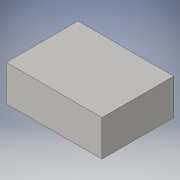
# Autodesk Inventor part: Brain
Saved by Autodesk Inventor 2016 (Build 200138000, 138)
## iProperties
Created: 2015-10-30
Part Number: Brain
Material: Generic
Document SubType Name: Modeling
Designer: rossmosier
Density: 1 g/cm^3
Appearance: Default
Author: rossmosier
Autodesk Inventor part; units mm, degrees
ref_plane "YZ Plane" through (0, 0, 0) normal (1, 0, 0) x (0, 1, 0)
ref_plane "XZ Plane" through (0, 0, 0) normal (0, 1, 0) x (-1, 0, 0)
ref_plane "XY Plane" through (0, 0, 0) normal (0, 0, 1) x (1, 0, 0)
sketch "Sketch1" plane through (0, 0, 0) normal (0, 1, 0) x (-1, 0, 0)
  line L0 (0, 0) -> (-203.2, 0)
  line L1 (-203.2, 0) -> (-203.2, -152.4)
  line L2 (-203.2, -152.4) -> (0, -152.4)
  line L3 (0, -152.4) -> (0, 0)
  dimension "d0" = 203.2
  dimension "d1" = 152.4
  constraints: 8 end point, 2 parallel, 1 horizontal, 1 perpendicular
  measures "d0" distance of L2.end L1.end
  measures "d1" distance of L1.end L0.end
extrude "Extrusion1" add sketch "Sketch1" along normal blind 76.2
sketch "Sketch2" plane through (0, 76.2, 0) normal (0, 1, 0) x (1, 0, 0)
  line L0 (0, 0) -> (203.2, 0) projected
  line L1 (203.2, 0) -> (203.2, 152.4) projected
  line L2 (203.2, 152.4) -> (0, 152.4) projected
  line L3 (0, 152.4) -> (0, 0) projected
  line L4 (203.2, 0) -> (101.6, 0) construction
  line L5 (101.6, 63.5) -> (203.2, 63.5) construction
  line L6 (203.2, 63.5) -> (203.2, 0) construction
  line L7 (203.2, 152.4) -> (101.6, 152.4) construction
  line L8 (101.6, 88.9) -> (203.2, 88.9) construction
  line L9 (203.2, 88.9) -> (203.2, 152.4) construction
  line L10 (0, 0) -> (203.2, 0) construction
  line L11 (203.2, 152.4) -> (0, 152.4) construction
  point P0 (101.6, 120.65)
  point P1 (101.6, 31.75)
  dimension "d4" = 101.6
  dimension "d5" = 63.5
  dimension "d6" = 101.6
  dimension "d7" = 63.5
  constraints: 12 end point, 2 horizontal, 2 parallel
  measures "d4" distance of L5.start L5.end
  measures "d5" distance of L4.end L5.start
  measures "d6" distance of L8.end L8.start
  measures "d7" distance of L8.start L7.end
sketch "Sketch3" plane through (0, 76.2, 0) normal (0, 1, 0) x (1, 0, 0)
  line L0 (0, 0) -> (203.2, 0) projected
  line L1 (203.2, 0) -> (203.2, 152.4) construction
  line L2 (203.2, 152.4) -> (0, 152.4) projected
  line L3 (0, 152.4) -> (0, 0) projected
  line L4 (203.2, 0) -> (203.2, 34.671) construction
  line L5 (203.2, 0) -> (203.2, 152.4) construction
  point P0 (152.4, 34.671)
  dimension "d10" = 34.671
  constraints: 2 end point, 1 point on line
  measures "d10" distance of L0.end L4.end
body "Solid1"
